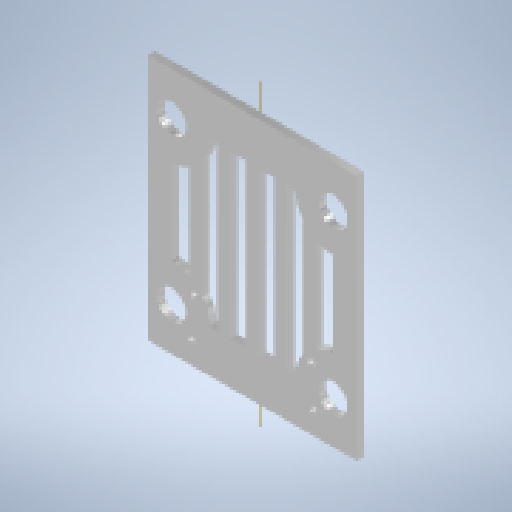
# Autodesk Inventor part: board_setter_base
Saved by Autodesk Inventor 2024.1 (Build 281209000, 209)
## iProperties
Created: 2024-10-09
Part Number: board_setter_base
Material: アルミニウム 6061
Document SubType Name: Sheet Metal
Designer: hibik
Density: 2.7 g/cm^3
Sheet Metal Rule: Default_mm
Appearance: アルミニウム - フラット
Author: hibik
Autodesk Inventor part; units mm, degrees
ref_plane "YZ Plane" through (0, 0, 0) normal (1, 0, 0) x (0, 1, 0)
ref_plane "XZ Plane" through (0, 0, 0) normal (0, 1, 0) x (-1, 0, 0)
ref_plane "XY Plane" through (0, 0, 0) normal (0, 0, 1) x (1, 0, 0)
sketch "スケッチ1" plane through (0, 0, 0) normal (0, 0, 1) x (1, 0, 0)
  line L0 (-22, -24) -> (22, -24)
  line L1 (22, -24) -> (22, 24)
  line L2 (22, 24) -> (-22, 24)
  line L3 (-22, 24) -> (-22, -24)
  line L4 (-22, -24) -> (22, 24) construction
  line L5 (22, -24) -> (-22, 24) construction
  line L6 (-17, 15) -> (17, 15)
  line L7 (17, 15) -> (17, -19)
  line L8 (17, -19) -> (-17, -19)
  line L9 (-17, -19) -> (-17, 15)
  circle A0 centre (-17, 15) radius 3
  circle A1 centre (17, 15) radius 3
  circle A2 centre (17, -19) radius 3
  circle A3 centre (-17, -19) radius 3
  circle A4 centre (-17, 15) radius 8
  circle A5 centre (17, 15) radius 8
  circle A6 centre (17, -19) radius 8
  circle A7 centre (-17, -19) radius 8
  line L10 (-22, -24) -> (22, -24)
  line L11 (22, -24) -> (22, -28)
  line L12 (22, -28) -> (-22, -28)
  line L13 (-22, -28) -> (-22, -24)
  line L14 (-1.5, 15) -> (1.5, 15)
  line L15 (1.5, 15) -> (1.5, -19)
  line L16 (1.5, -19) -> (-1.5, -19)
  line L17 (-1.5, -19) -> (-1.5, 15)
  line L18 (7.5, 15) -> (7.5, -19)
  line L19 (4.5, -19) -> (4.5, 15)
  line L20 (13.5, 15) -> (13.5, -19)
  line L21 (10.5, -19) -> (10.5, 15)
  line L22 (-4.5, 15) -> (-4.5, -19)
  line L23 (-7.5, -19) -> (-7.5, 15)
  line L24 (1.5, 15) -> (1.5, -19)
  line L25 (-1.5, -19) -> (-1.5, 15)
  line L26 (7.5, 15) -> (7.5, -19)
  line L27 (4.5, -19) -> (4.5, 15)
  line L28 (-10.5, 15) -> (-10.5, -19)
  line L29 (-13.5, -19) -> (-13.5, 15)
  line L30 (-4.5, 15) -> (-4.5, -19)
  line L31 (-7.5, -19) -> (-7.5, 15)
  line L32 (1.5, 15) -> (1.5, -19)
  line L33 (-1.5, -19) -> (-1.5, 15)
  point P0 (0, 0)
  point P1 (-9, 15)
  point P2 (9, 15)
  point P3 (17, 7)
  point P4 (17, -11)
  point P5 (9, -19)
  point P6 (-9, -19)
  point P7 (-17, -11)
  point P8 (-17, 7)
  point P9 (22, -24)
  point P10 (0, 15)
  point P11 (-13.5, 7.8063)
  point P12 (-13.5, -11.8063)
  point P13 (-10.5, -14.3363)
  point P14 (-10.5, 10.3363)
  point P15 (10.5, 10.3363)
  point P16 (10.5, -14.3363)
  point P17 (13.5, -11.8063)
  point P18 (13.5, 7.8063)
  dimension "d0" = 48
  dimension "d1" = 44
  dimension "d2" = 34
  dimension "d3" = 5
  dimension "d4" = 5
  dimension "d5" = 6
  dimension "d6" = 16
  dimension "d11" = 4
  dimension "d12" = 3
  dimension "d15" = 6
  dimension "d18" = 6
  measures "d0" distance of L2.end L0.start
  measures "d1" distance of L1.end L2.end
  measures "d2" distance of L7.end L8.end
  measures "d3" distance between parallel lines of L3 L9
  measures "d4" distance between parallel lines of L0 L8
  measures "d5" diameter of A0
  measures "d6" diameter of A4
  measures "d11" distance of L10.end L11.end
  measures "d12" distance between parallel lines of L15 L17
  measures "d15" distance of L14.end L18.start
  measures "d18" distance of L14.end L22.start
extrude "プレート1" add sketch "スケッチ1" along normal blind 1.5 contours L3 A7 L9 A3 L8 L0 | L0 A7 L13 | A7 L8 A6 L0 | L0 A6 L11 L12 L13 A7 | L3 A4 L9 A7 | A6 L8 A2 L7 L1 L0 | L0 L11 A6 | L8 L28 A7 | L3 A4 L6 A0 L9 | A7 L29 L8 A3 L9 | A6 L21 L8 | L23 L6 L22 L8 | L8 L29 A7 L28 | A7 L29 A4 L28 | L3 L2 L1 A5 L6 A4 | L9 A0 L6 L29 A4 | A6 L7 A5 L1 | L21 A6 L20 L8 | L8 L19 L6 L18 | L21 A5 L20 A6 | L28 L6 A4 | A4 L29 L6 L28 | A5 L7 A1 L6 L1 | L7 A2 L8 L20 A6 | L21 L6 L20 A5 | A5 L6 L21 | L17 L6 L15 L8 | A5 L20 L6 A1 L7
sketch "スケッチ2" plane through (0, 0, 1.5) normal (0, 0, 1) x (1, 0, 0)
  line L0 (11.5, -21.5) -> (11.5, -14.8) projected
  line L1 (11.5, -21.5) -> (12, -21.5) projected
  line L2 (12, -21.5) -> (12, -24) projected
  line L3 (18, -24) -> (14, -24) projected
  line L4 (18, -14) -> (18, -24) construction
  line L5 (12.3, -14) -> (18, -14) projected
  circle A0 centre (12.3, -14.8) radius 0.8
  circle A1 centre (14, -23.2) radius 0.8
  line L6 (0, 0) -> (0, -10)
  circle A2 centre (-12.3, -14.8) radius 0.8
  circle A3 centre (-14, -23.2) radius 0.8
  arc A4 (11.5, -14.8) -> (12.3, -14) centre (12.3, -14.8) ccw projected
  line L7 (14, -24) -> (12, -24) projected
  circle A5 centre (14, -23.2) radius 0.8 projected
  dimension "d21" = 1.6
  dimension "d22" = 1.6
  dimension "d25" = 2
  constraints: 4 centre point, 3 tangent, 2 end point, 2 symmetric about line, 1 vertical, 1 vertical alignment, 2 other
  measures "d21" diameter of A0
  measures "d22" diameter of A1
  measures "d25" distance from line of L2 A1.centre
extrude "切り取り1" cut sketch "スケッチ2" against normal blind 1.5
equation "\"d4\" = d3"
equation "\"d23\" = Thickness"
equation "\"d10\" = Thickness"
equation "\"BendRadius\" = Thickness"
equation "\"BendReliefWidth\" = Thickness"
equation "\"BendReliefDepth\" = 0.5 * Thickness"
equation "\"CornerReliefSize\" = 4 * Thickness"
equation "\"MinimumRemnant\" = 2 * Thickness"
equation "\"TransitionRadius\" = BendRadius"
equation "\"JacobiRadiusSize\" = BendRadius"
equation "\"GapSize\" = Thickness"
equation "\"Thickness\" = 1.5"
